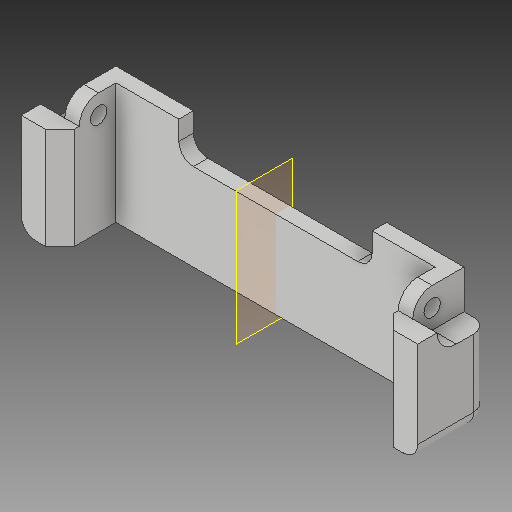
# Autodesk Inventor part: SwitchCov
Saved by Autodesk Inventor 2018 (Build 220112000, 112)
## iProperties
Created: 2017-07-28
Part Number: SwitchCov
Material: 一般
Document SubType Name: Modeling
Designer: g45k
Density: 1 g/cm^3
Appearance: 既定
Author: g45k
Autodesk Inventor part; units mm, degrees
ref_plane "YZ Plane" through (0, 0, 0) normal (1, 0, 0) x (0, 1, 0)
ref_plane "XZ Plane" through (0, 0, 0) normal (0, 1, 0) x (-1, 0, 0)
ref_plane "XY Plane" through (0, 0, 0) normal (0, 0, 1) x (1, 0, 0)
sketch "スケッチ1" plane through (0, 0, 0) normal (0, 0, 1) x (1, 0, 0)
  line L0 (-24.1162, 3.8741) -> (41.8838, 3.8741)
  line L1 (41.8838, 3.8741) -> (41.8838, -21.1259)
  line L2 (41.8838, -21.1259) -> (-24.1162, -21.1259)
  line L3 (-24.1162, -21.1259) -> (-24.1162, 3.8741)
  point P0 (0, 0)
  dimension "d0" = 66
  dimension "d1" = 25
  constraints: 8 end point, 2 parallel, 1 horizontal, 1 perpendicular
  measures "d0" distance of L1.end L2.end
  measures "d1" distance of L0.end L1.end
extrude "押し出し1" add sketch "スケッチ1" along normal blind 3
sketch "スケッチ2" plane through (41.8838, -21.1259, 0) normal (1, 0, 0) x (0, 0, -1)
  line L0 (0, 25) -> (-3, 25) construction
  line L1 (0, 25) -> (0, 0) construction
  line L2 (-3, 0) -> (-3, 25) construction
  line L3 (0, 25) -> (-10.6, 25)
  line L4 (-10.6, 25) -> (-10.6, 17)
  line L5 (-10.6, 17) -> (0, 17)
  line L6 (0, 17) -> (0, 25)
  circle A0 centre (-6.6, 21) radius 1.7
  dimension "d4" = 8
  dimension "d5" = 3.4
  dimension "d6" = 3.6
  dimension "d7" = 4
  dimension "d8" = 4
  constraints: 8 end point, 2 parallel, 1 centre point, 1 horizontal, 1 perpendicular
  measures "d4" distance of L4.end L3.end
  measures "d5" diameter of A0
  measures "d6" distance from line of L2 A0.centre
  measures "d7" distance from line of L3 A0.centre
  measures "d8" distance from line of A0.centre L4
extrude "押し出し2" add sketch "スケッチ2" along normal blind 3
fillet "フィレット1" radius 4 2 edges at (43.3838, 3.8741, 10.6) (43.3838, -4.1259, 10.6)
sketch "スケッチ3" plane through (41.8838, -21.1259, 3) normal (1, 0, 0) x (0, 0, -1)
  line L0 (3, 17) -> (0, 17) construction
  line L1 (3, 17) -> (3, 0) construction
  line L2 (-3.6, 17) -> (0, 17) construction
  line L3 (-3.6, 17) -> (3, 17)
  line L4 (3, 17) -> (3, 0)
  line L5 (3, 0) -> (-3.6, 0)
  line L6 (-3.6, 0) -> (-3.6, 17)
  line L7 (3, 0) -> (0, 0) construction
  constraints: 8 end point, 2 parallel, 1 collinear, 1 horizontal, 1 perpendicular, 1 point on line
extrude "押し出し3" add sketch "スケッチ3" along normal blind 8
sketch "スケッチ4" plane through (0, 0, 3) normal (0, 0, 1) x (1, 0, 0)
  line L0 (41.8838, 3.8741) -> (-24.1162, 3.8741) construction
  line L1 (8.8838, 3.8741) -> (8.8838, 19.0271) construction
  line L2 (-24.1162, 3.8741) -> (44.8838, 3.8741) projected
  line L3 (28.8838, 3.8741) -> (-11.1162, 3.8741)
  line L4 (-11.1162, 3.8741) -> (-11.1162, -3.1259)
  line L5 (-11.1162, -3.1259) -> (28.8838, -3.1259)
  line L6 (28.8838, -3.1259) -> (28.8838, 3.8741)
  dimension "d15" = 40
  dimension "d16" = 7
  constraints: 10 end point, 2 parallel, 1 horizontal, 1 midpoint, 1 perpendicular, 1 point on line, 1 vertical, 1 other
  measures "d15" distance between parallel lines of L4 L6
  measures "d16" distance of L5.end L3.start
extrude "押し出し4" cut sketch "スケッチ4" against normal blind 5
sketch "スケッチ5" plane through (41.8838, -21.1259, 0) normal (-1, 0, 0) x (0, 0, 1)
  line L0 (6.6, 0) -> (6.6, 17) construction
  line L1 (6.6, 0) -> (14.6, 0)
  line L2 (14.6, 0) -> (14.6, 21)
  line L3 (14.6, 21) -> (10.6, 21)
  line L4 (6.6, 17) -> (6.6, 0)
  arc A0 (6.6, 17) -> (10.6, 21) centre (6.6, 21) ccw
  arc A1 (6.6, 17) -> (6.6, 25) centre (6.6, 21) ccw projected
  line L5 (6.6, 0) -> (6.6, 17) projected
  line L6 (3, 0) -> (6.6, 0) projected
  dimension "d26" = 8
  constraints: 10 end point, 3 point on circle, 2 collinear, 2 parallel, 1 centre point, 1 coincident, 1 concentric, 1 horizontal, 1 perpendicular, 1 point on line
  measures "d26" distance of L0.start L1.end
extrude "押し出し5" add sketch "スケッチ5" against normal up to surface (8 mm away)
chamfer "面取り2" distance 3 angle 45 1 edges at (41.8838, -10.6259, 14.6)
ref_plane "作業平面1" through (8.8838, 3.8741, 3) normal (1, 0, 0) x (0, 0, -1)
mirror "ミラー3" about plane through (8.8838, 3.8741, 3) normal (1, 0, 0) of "押し出し2", "フィレット1", "押し出し3", "押し出し5", "面取り2"
fillet "フィレット3" radius 3 8 edges at (49.8838, -21.1259, 7.3) (49.8838, -12.6259, 0) (8.8838, -21.1259, 0) (-32.1162, -21.1259, 10.6) (-32.1162, -21.1259, 3.3) (-32.1162, -12.6259, 0) (-11.1162, -3.1259, 1.5) (28.8838, -3.1259, 1.5)
